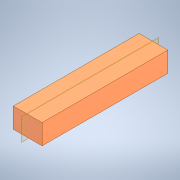
# Autodesk Inventor part: Contenedor3
Saved by Autodesk Inventor 2020.3 (Build 243373000, 373)
## iProperties
Created: 2020-09-22
Part Number: Contenedor3
Material: ABS Plastic
Document SubType Name: Modeling
Designer: juanp
Density: 1.06 g/cm^3
Appearance: Smooth - White
Author: juanp
Autodesk Inventor part; units mm, degrees
ref_plane "YZ Plane" through (0, 0, 0) normal (1, 0, 0) x (0, 1, 0)
ref_plane "XZ Plane" through (0, 0, 0) normal (0, 1, 0) x (-1, 0, 0)
ref_plane "XY Plane" through (0, 0, 0) normal (0, 0, 1) x (1, 0, 0)
sketch "Sketch1" plane through (0, 0, 0) normal (0, 1, 0) x (-1, 0, 0)
  line L0 (0, 0) -> (0, -358.09) construction
  line L1 (42, 13.5039) -> (0, 13.5039)
  line L2 (0, 13.5039) -> (0, -13.5039)
  line L3 (0, -13.5039) -> (42, -13.5039)
  line L4 (42, -13.5039) -> (42, 13.5039)
  line L5 (42, -15.5039) -> (0, -15.5039)
  line L6 (0, -15.5039) -> (0, -42.5117)
  line L7 (0, -42.5117) -> (42, -42.5117)
  line L8 (42, -42.5117) -> (42, -15.5039)
  line L9 (42, -44.5117) -> (0, -44.5117)
  line L10 (0, -44.5117) -> (0, -71.5196)
  line L11 (0, -71.5196) -> (42, -71.5196)
  line L12 (42, -71.5196) -> (42, -44.5117)
  line L13 (42, -104.5274) -> (0, -104.5274)
  line L14 (0, -104.5274) -> (0, -131.5352)
  line L15 (0, -131.5352) -> (42, -131.5352)
  line L16 (42, -131.5352) -> (42, -104.5274)
  line L17 (42, -133.5352) -> (0, -133.5352)
  line L18 (0, -133.5352) -> (0, -160.543)
  line L19 (0, -160.543) -> (42, -160.543)
  line L20 (42, -160.543) -> (42, -133.5352)
  line L21 (42, -75.5196) -> (0, -75.5196)
  line L22 (0, -75.5196) -> (0, -102.5274)
  line L23 (0, -102.5274) -> (42, -102.5274)
  line L24 (42, -102.5274) -> (42, -75.5196)
  line L25 (21, -13.5039) -> (21, -15.5039)
  line L26 (21, -42.5117) -> (21, -44.5117)
  line L27 (21, -102.5274) -> (21, -104.5274)
  line L28 (21, -131.5352) -> (21, -133.5352)
  line L29 (42, -164.543) -> (0, -164.543)
  line L30 (0, -164.543) -> (0, -191.5509)
  line L31 (0, -191.5509) -> (42, -191.5509)
  line L32 (42, -191.5509) -> (42, -164.543)
  line L33 (42, -193.5509) -> (0, -193.5509)
  line L34 (0, -193.5509) -> (0, -220.5587)
  line L35 (0, -220.5587) -> (42, -220.5587)
  line L36 (42, -220.5587) -> (42, -193.5509)
  line L37 (42, -222.5587) -> (0, -222.5587)
  line L38 (0, -222.5587) -> (0, -249.5665)
  line L39 (0, -249.5665) -> (42, -249.5665)
  line L40 (42, -249.5665) -> (42, -222.5587)
  line L41 (42, -282.5743) -> (0, -282.5743)
  line L42 (0, -282.5743) -> (0, -309.5822)
  line L43 (0, -309.5822) -> (42, -309.5822)
  line L44 (42, -309.5822) -> (42, -282.5743)
  line L45 (42, -311.5822) -> (0, -311.5822)
  line L46 (0, -311.5822) -> (0, -338.59)
  line L47 (0, -338.59) -> (42, -338.59)
  line L48 (42, -338.59) -> (42, -311.5822)
  line L49 (42, -253.5665) -> (0, -253.5665)
  line L50 (0, -253.5665) -> (0, -280.5743)
  line L51 (0, -280.5743) -> (42, -280.5743)
  line L52 (42, -280.5743) -> (42, -253.5665)
  line L53 (21, -191.5509) -> (21, -193.5509)
  line L54 (21, -220.5587) -> (21, -222.5587)
  line L55 (21, -280.5743) -> (21, -282.5743)
  line L56 (21, -309.5822) -> (21, -311.5822)
  line L57 (21, -338.59) -> (21, -340.59)
  line L58 (88, 15.5039) -> (-2, 15.5039)
  line L59 (-2, 15.5039) -> (-2, -377.59)
  line L60 (-2, -377.59) -> (88, -377.59)
  line L61 (88, -377.59) -> (88, 15.5039)
  line L62 (44, 0) -> (44, -358.09) construction
  line L63 (86, 13.5039) -> (44, 13.5039)
  line L64 (44, 13.5039) -> (44, -13.5039)
  line L65 (44, -13.5039) -> (86, -13.5039)
  line L66 (86, -13.5039) -> (86, 13.5039)
  line L67 (86, -15.5039) -> (44, -15.5039)
  line L68 (44, -15.5039) -> (44, -42.5117)
  line L69 (44, -42.5117) -> (86, -42.5117)
  line L70 (86, -42.5117) -> (86, -15.5039)
  line L71 (86, -44.5117) -> (44, -44.5117)
  line L72 (44, -44.5117) -> (44, -71.5196)
  line L73 (44, -71.5196) -> (86, -71.5196)
  line L74 (86, -71.5196) -> (86, -44.5117)
  line L75 (86, -104.5274) -> (44, -104.5274)
  line L76 (44, -104.5274) -> (44, -131.5352)
  line L77 (44, -131.5352) -> (86, -131.5352)
  line L78 (86, -131.5352) -> (86, -104.5274)
  line L79 (86, -133.5352) -> (44, -133.5352)
  line L80 (44, -133.5352) -> (44, -160.543)
  line L81 (44, -160.543) -> (86, -160.543)
  line L82 (86, -160.543) -> (86, -133.5352)
  line L83 (86, -75.5196) -> (44, -75.5196)
  line L84 (44, -75.5196) -> (44, -102.5274)
  line L85 (44, -102.5274) -> (86, -102.5274)
  line L86 (86, -102.5274) -> (86, -75.5196)
  line L87 (65, -13.5039) -> (65, -15.5039)
  line L88 (65, -42.5117) -> (65, -44.5117)
  line L89 (65, -102.5274) -> (65, -104.5274)
  line L90 (65, -131.5352) -> (65, -133.5352)
  line L91 (44, -222.5587) -> (44, -249.5665)
  line L92 (86, -249.5665) -> (86, -222.5587)
  line L93 (86, -253.5665) -> (44, -253.5665)
  line L94 (44, -253.5665) -> (44, -280.5743)
  line L95 (86, -280.5743) -> (86, -253.5665)
  line L96 (44, -249.5665) -> (86, -249.5665)
  line L97 (86, -164.543) -> (44, -164.543)
  line L98 (44, -164.543) -> (44, -191.5509)
  line L99 (44, -191.5509) -> (86, -191.5509)
  line L100 (86, -191.5509) -> (86, -164.543)
  line L101 (86, -222.5587) -> (44, -222.5587)
  line L102 (65, -220.5587) -> (65, -222.5587)
  line L103 (44, -220.5587) -> (86, -220.5587)
  line L104 (86, -220.5587) -> (86, -193.5509)
  line L105 (86, -193.5509) -> (44, -193.5509)
  line L106 (44, -193.5509) -> (44, -220.5587)
  line L107 (65, -191.5509) -> (65, -193.5509)
  line L108 (86, -282.5743) -> (44, -282.5743)
  line L109 (44, -282.5743) -> (44, -309.5822)
  line L110 (44, -309.5822) -> (86, -309.5822)
  line L111 (86, -309.5822) -> (86, -282.5743)
  line L112 (44, -280.5743) -> (86, -280.5743)
  line L113 (65, -309.5822) -> (65, -311.5822)
  line L114 (86, -311.5822) -> (44, -311.5822)
  line L115 (86, -338.59) -> (86, -311.5822)
  line L116 (44, -338.59) -> (86, -338.59)
  line L117 (44, -311.5822) -> (44, -338.59)
  line L118 (65, -280.5743) -> (65, -282.5743)
  line L119 (65, 13.5039) -> (65, 15.5039)
  line L120 (65, -71.5196) -> (65, -75.5196)
  line L121 (21, -71.5196) -> (21, -75.5196)
  line L122 (65, -160.543) -> (65, -164.543)
  line L123 (21, -160.543) -> (21, -164.543)
  line L124 (65, -249.5665) -> (65, -253.5665)
  line L125 (21, -249.5665) -> (21, -253.5665)
  line L126 (0, -340.59) -> (86, -340.59)
  line L127 (86, -340.59) -> (86, -375.59)
  line L128 (86, -375.59) -> (0, -375.59)
  line L129 (0, -375.59) -> (0, -340.59)
  line L130 (65, -338.59) -> (65, -340.59)
  line L131 (86, -358.09) -> (0, -358.09) construction
  point P0 (0, -29.0078)
  point P1 (0, -58.0157)
  point P2 (0, -118.0313)
  point P3 (0, -147.0391)
  point P4 (0, -89.0235)
  point P5 (0, -178.047)
  point P6 (0, -207.0548)
  point P7 (0, -236.0626)
  point P8 (0, -296.0783)
  point P9 (0, -325.0861)
  point P10 (0, -267.0704)
  point P11 (44, -29.0078)
  point P12 (44, -58.0157)
  point P13 (44, -118.0313)
  point P14 (44, -147.0391)
  point P15 (44, -89.0235)
  point P16 (44, -236.0626)
  point P17 (44, -267.0704)
  point P18 (44, -178.047)
  point P19 (44, -207.0548)
  point P20 (44, -296.0783)
  point P21 (44, -325.0861)
  dimension "d0" = 358.09
  dimension "d7" = 2
  dimension "d8" = 2
  dimension "d10" = 358.09
  dimension "d12" = 2
  dimension "d13" = 2
  dimension "d14" = 90
  dimension "d15" = 2
  dimension "d16" = 4
  dimension "d17" = 4
  dimension "d18" = 4
  dimension "d24" = 2
  dimension "d25" = 35
  constraints: 260 end point, 73 midpoint, 66 equal length, 52 parallel, 28 perpendicular, 26 horizontal, 4 point on line, 1 collinear, 1 vertical, 29 other
  measures "d0" distance of point (0, 0) point (0, -358.09)
  measures "d7" distance between parallel lines of L59 L2
  measures "d8" distance between parallel lines of L58 L1
  measures "d10" distance of point (44, 0) point (44, -358.09)
  measures "d12" distance of L119.start L119.end
  measures "d13" distance between parallel lines of L61 L74
  measures "d14" distance of L59.end L60.end
  measures "d15" distance between parallel lines of L4 L64
  measures "d16" distance of L121.start L121.end
  measures "d17" distance of L123.start L123.end
  measures "d18" distance of L125.start L125.end
  measures "d24" distance between parallel lines of L60 L128
  measures "d25" distance of L126.end L127.end
extrude "Extrusion1" add sketch "Sketch1" along normal blind 60
sketch "Sketch2" plane through (0, 60, 0) normal (0, 1, 0) x (1, 0, 0)
  line L0 (2, -15.5039) -> (2, 377.59) projected
  line L1 (-88, -15.5039) -> (2, -15.5039) projected
  line L2 (-88, 377.59) -> (-88, -15.5039) projected
  line L3 (2, 377.59) -> (-88, 377.59) projected
  point P0 (0, 0)
extrude "Extrusion2" add sketch "Sketch2" along normal blind 3
fillet "Fillet1" radius 5 192 edges at (-42, 30, -44.5117) (0, 30, -44.5117) (-42, 30, -42.5117) (0, 30, -15.5039) (-21, 60, 13.5039) (-44, 30, -102.5274) (-44, 30, -104.5274) (-44, 30, -131.5352) (-86, 30, -131.5352) (-86, 30, -104.5274) (-86, 30, -75.5196) (0, 30, -71.5196) (-21, 60, -42.5117) (-86, 30, -13.5039) (-86, 30, -15.5039) (-44, 30, -15.5039) (-86, 30, 13.5039) (-44, 30, -13.5039) (-44, 30, 13.5039) (-42, 30, -15.5039) (-86, 60, -267.0704) (-42, 60, -296.0783) (-65, 60, -282.5743) (-86, 60, -296.0783) (-44, 60, -296.0783) (-42, 60, -267.0704) (-44, 60, -267.0704) (-42, 60, -236.0626) (-65, 60, -280.5743) (-65, 60, -309.5822) (0, 30, -42.5117) (-42, 60, -29.0078) (-21, 60, -15.5039) (-42, 30, -13.5039) (0, 30, -13.5039) (0, 30, 13.5039) (0, 30, -160.543) (0, 30, -133.5352) (0, 30, -131.5352) (-42, 30, -160.543) (-42, 30, -133.5352) (-86, 30, -133.5352) (-44, 30, -133.5352) (-86, 30, -160.543) (-44, 30, -160.543) (-86, 30, -164.543) (-44, 60, -178.047) (0, 30, -191.5509) (-42, 30, -164.543) (-42, 30, -191.5509) (0, 30, -164.543) (-44, 30, -42.5117) (-44, 30, -44.5117) (-44, 30, -71.5196) (-44, 30, -75.5196) (-86, 30, -42.5117) (-86, 30, -44.5117) (-21, 60, -13.5039) (-86, 30, -71.5196) (-42, 30, 13.5039) (-86, 30, -102.5274) (-65, 60, -220.5587) (-86, 60, -207.0548) (-65, 60, -193.5509) (-44, 60, -207.0548) (-65, 60, -164.543) (-65, 60, -191.5509) (-86, 60, -178.047) (-65, 60, -160.543) (-44, 30, -164.543) (-86, 30, -191.5509) (-86, 30, -193.5509) (-86, 30, -220.5587) (-44, 30, -220.5587) (-44, 30, -191.5509) (0, 30, -220.5587) (0, 30, -193.5509) (-42, 30, -193.5509) (-42, 30, -220.5587) (-42, 60, -178.047) (0, 60, -178.047) (-21, 60, -193.5509) (-21, 60, -220.5587) (-42, 60, -207.0548) (0, 60, -207.0548) (-21, 60, -222.5587) (0, 60, -236.0626) (-21, 60, -191.5509) (-44, 30, -193.5509) (-86, 30, -222.5587) (-44, 30, -222.5587) (-86, 30, -249.5665) (-44, 30, -249.5665) (-86, 30, -253.5665) (-65, 60, -253.5665) (-65, 60, -249.5665) (-86, 60, -236.0626) (-44, 60, -236.0626) (-65, 60, -222.5587) (0, 30, -249.5665) (0, 30, -222.5587) (-42, 30, -249.5665) (-42, 30, -222.5587) (-86, 30, -280.5743) (0, 30, -309.5822) (0, 30, -282.5743) (-42, 30, -282.5743) (-42, 30, -309.5822) (-44, 30, -253.5665) (-44, 30, -280.5743) (-44, 30, -282.5743) (-44, 30, -309.5822) (-86, 30, -309.5822) (-86, 30, -282.5743) (-42, 30, -311.5822) (-42, 30, -338.59) (0, 30, -311.5822) (-44, 30, -311.5822) (-86, 30, -311.5822) (-44, 30, -338.59) (-86, 30, -338.59) (0, 30, -338.59) (-21, 60, -249.5665) (-21, 60, -253.5665) (0, 60, -267.0704) (-21, 60, -280.5743) (0, 60, -296.0783) (-21, 60, -282.5743) (-21, 60, -309.5822) (-21, 60, -311.5822) (-65, 60, -311.5822) (-42, 60, -325.0861) (-21, 60, -338.59) (0, 60, -325.0861) (-44, 60, -325.0861) (-86, 60, -325.0861) (-65, 60, -338.59) (0, 30, -280.5743) (0, 30, -253.5665) (-42, 30, -253.5665) (-42, 30, -280.5743) (-65, 60, -71.5196) (-86, 60, -58.0157) (-65, 60, -44.5117) (-44, 60, -58.0157) (-65, 60, -42.5117) (-86, 60, -29.0078) (-65, 60, -15.5039) (-44, 60, -29.0078) (-65, 60, -13.5039) (-86, 60, 0) (-65, 60, 13.5039) (-44, 60, 0) (-44, 60, -147.0391) (-86, 60, -147.0391) (-65, 60, -131.5352) (-65, 60, -133.5352) (-86, 60, -118.0313) (-44, 60, -118.0313) (-65, 60, -104.5274) (-21, 60, -131.5352) (-21, 60, -133.5352) (0, 60, -147.0391) (-21, 60, -160.543) (-42, 60, -147.0391) (-21, 60, -104.5274) (0, 60, -118.0313) (-42, 60, -118.0313) (-21, 60, -102.5274) (-21, 60, -75.5196) (-42, 60, -89.0235) (0, 60, -89.0235) (-21, 60, -164.543) (-42, 30, -71.5196) (-42, 30, -131.5352) (0, 30, -104.5274) (-42, 30, -104.5274) (0, 30, -102.5274) (-42, 30, -102.5274) (-21, 60, -44.5117) (0, 60, -58.0157) (-42, 60, -58.0157) (-21, 60, -71.5196) (0, 60, -29.0078) (-42, 60, 0) (0, 60, 0) (0, 30, -75.5196) (-42, 30, -75.5196) (-86, 60, -89.0235) (-65, 60, -75.5196) (-44, 60, -89.0235) (-65, 60, -102.5274)
ref_plane "Work Plane1" through (-88, 0, -181.043) normal (0, 0, 1) x (1, 0, 0)
ref_plane "Work Plane2" through (-43, 0, 15.5039) normal (1, 0, 0) x (0, 0, -1)
body "Solid1"
